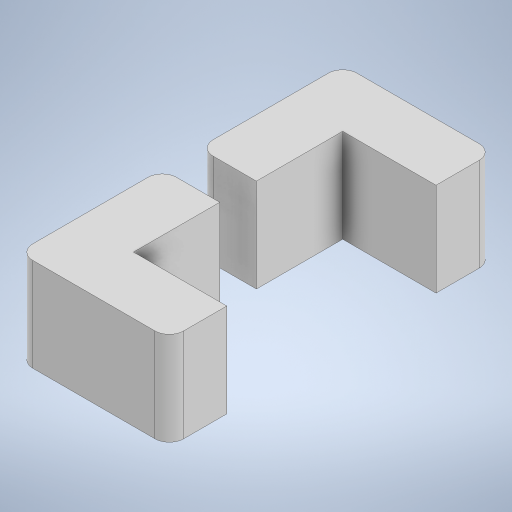
# Autodesk Inventor part: BH_MK1
Saved by Autodesk Inventor 2024 (Build 280153000, 153)
## iProperties
Created: 2023-08-02
Part Number: BH_MK1
Material: Generic
Document SubType Name: Modeling
Designer: s137416
Density: 1 g/cm^3
Appearance: Default
Author: s137416
Autodesk Inventor part; units mm, degrees
ref_plane "YZ Plane" through (0, 0, 0) normal (1, 0, 0) x (0, 1, 0)
ref_plane "XZ Plane" through (0, 0, 0) normal (0, 1, 0) x (-1, 0, 0)
ref_plane "XY Plane" through (0, 0, 0) normal (0, 0, 1) x (1, 0, 0)
sketch "Sketch1" plane through (0, 0, 0) normal (0, 1, 0) x (-1, 0, 0)
  line L0 (-82.55, 88.9) -> (82.55, 88.9)
  line L1 (82.55, 88.9) -> (82.55, -88.9)
  line L2 (82.55, -88.9) -> (-82.55, -88.9)
  line L3 (-82.55, -88.9) -> (-82.55, 88.9)
  line L4 (-82.55, 88.9) -> (82.55, -88.9) construction
  line L5 (82.55, 88.9) -> (-82.55, -88.9) construction
  line L6 (5.6683, 92.4026) -> (107.2683, 92.4026)
  line L7 (107.2683, 92.4026) -> (107.2683, 143.2026)
  line L8 (107.2683, 143.2026) -> (5.6683, 143.2026)
  line L9 (5.6683, 143.2026) -> (5.6683, 92.4026)
  line L10 (138.926, 16.2026) -> (88.126, 16.2026)
  line L11 (88.126, 16.2026) -> (88.126, 143.2026)
  line L12 (88.126, 143.2026) -> (138.926, 143.2026)
  line L13 (138.926, 143.2026) -> (138.926, 16.2026)
  line L14 (5.6683, -92.4026) -> (107.2683, -92.4026)
  line L15 (107.2683, -92.4026) -> (107.2683, -143.2026)
  line L16 (107.2683, -143.2026) -> (5.6683, -143.2026)
  line L17 (5.6683, -143.2026) -> (5.6683, -92.4026)
  line L18 (88.126, -143.2026) -> (138.926, -143.2026)
  line L19 (138.926, -143.2026) -> (138.926, -16.2026)
  line L20 (138.926, -16.2026) -> (88.126, -16.2026)
  line L21 (88.126, -16.2026) -> (88.126, -143.2026)
  point P0 (0, 0)
  point P1 (88.126, -92.4026)
  point P2 (88.126, 92.4026)
  dimension "d0" = 165.1
  dimension "d1" = 177.8
  dimension "d2" = 101.6
  dimension "d3" = 50.8
  dimension "d4" = 50.8
  dimension "d5" = 19.1423
  dimension "d6" = 3.5026
  dimension "d7" = 3.5026
  dimension "d8" = 101.6
  dimension "d9" = 50.8
  dimension "d10" = 50.8
  dimension "d11" = 0
  dimension "d12" = 127
  dimension "d13" = 127
  constraints: 44 end point, 10 parallel, 5 horizontal, 5 perpendicular, 2 midpoint, 2 point on line
  measures "d0" distance of L1.end L2.end
  measures "d1" distance of L0.end L1.end
  measures "d2" distance of L8.end L7.end
  measures "d3" distance of L6.end L7.end
  measures "d4" distance of L10.start L10.end
  measures "d5" distance between parallel lines of L11 L7
  measures "d6" distance between parallel lines of L6 L0
  measures "d7" distance between parallel lines of L2 L14
  measures "d8" distance of L15.end L16.end
  measures "d9" distance of L14.end L15.end
  measures "d10" distance of L20.end L19.end
  measures "d11" distance between parallel lines of L19 L13
  measures "d12" distance of L12.end L10.start
  measures "d13" distance of L18.end L19.end
extrude "Extrusion1" add sketch "Sketch1" along normal blind 82.55 contours L9 L8 L11 L6 | L11 L8 L7 L6 | L6 L7 L12 L13 L10 L11 | L14 L21 L16 L17 | L21 L20 L19 L18 L15 L14 | L14 L15 L16 L21
fillet "Fillet1" radius 12.7 1 edges at (-138.926, 41.275, 143.2026)
fillet "Fillet2" radius 12.7 3 edges at (-138.926, 41.275, -143.2026) (-5.6683, 41.275, 143.2026) (-5.6683, 41.275, -143.2026)
fillet "Fillet3" radius 12.7 2 edges at (-138.926, 41.275, -16.2026) (-138.926, 41.275, 16.2026)
body "Solid1"
